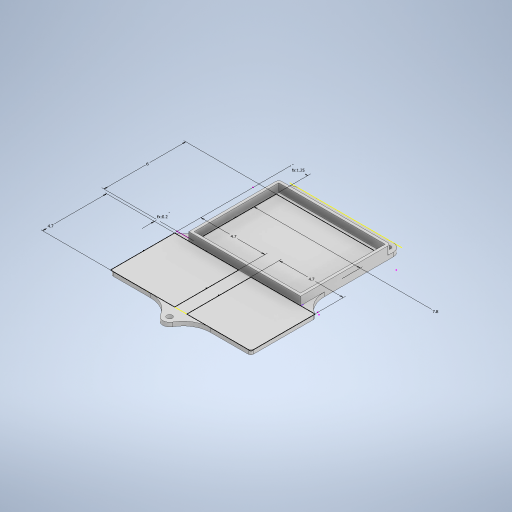
# Autodesk Inventor part: baseCarrito2
Saved by Autodesk Inventor 2024 (Build 280153000, 153)
## iProperties
Created: 2024-04-22
Part Number: baseCarrito2
Material: Generic
Document SubType Name: Modeling
Designer: Ruki
Density: 1 g/cm^3
Appearance: Default
Author: Ruki
Autodesk Inventor part; units mm, degrees
ref_plane "YZ Plane" through (0, 0, 0) normal (1, 0, 0) x (0, 1, 0)
ref_plane "XZ Plane" through (0, 0, 0) normal (0, 1, 0) x (-1, 0, 0)
ref_plane "XY Plane" through (0, 0, 0) normal (0, 0, 1) x (1, 0, 0)
sketch "Sketch1" plane through (0, 0, 0) normal (0, 1, 0) x (-1, 0, 0)
  line L0 (0, 0) -> (-103, 0)
  line L1 (-103, 0) -> (-103, -121)
  line L2 (-103, -121) -> (0, -121)
  line L3 (0, -121) -> (0, 0)
  line L4 (-10.5, -121) -> (-92.5, -121)
  line L5 (-92.5, -121) -> (-92.5, -49)
  line L6 (-92.5, -49) -> (-10.5, -49)
  line L7 (-10.5, -49) -> (-10.5, -121)
  circle A0 centre (-15.5, -116) radius 2
  circle A1 centre (-87.5, -116) radius 2
  line L8 (0, -49) -> (-47, -49)
  line L9 (-47, -49) -> (-47, -2)
  line L10 (-47, -2) -> (0, -2)
  line L11 (0, -2) -> (0, -49)
  line L12 (-56, -49) -> (-103, -49)
  line L13 (-103, -49) -> (-103, -2)
  line L14 (-103, -2) -> (-56, -2)
  line L15 (-56, -2) -> (-56, -49)
  line L16 (-10.5, -49) -> (0, -49)
  line L17 (-92.5, -49) -> (-103, -49)
  circle A2 centre (-51.5, 8) radius 2
  circle A3 centre (-51.5, 8) radius 5
  line L18 (-46.5, 8) -> (-46.5, 0)
  line L19 (-46.5, 0) -> (-56.5, 0)
  line L20 (-56.5, 0) -> (-56.5, 8)
  line L21 (0, -47) -> (-103, -47)
  line L22 (-10.5, -49) -> (-10.5, -47)
  line L23 (-92.5, -49) -> (-92.5, -47)
  point P0 (0, -62)
  point P1 (-103, -62)
  point P2 (-51.5, -121)
  point P3 (-92.5, -121)
  point P4 (-10.5, -121)
  point P5 (0, -25.5)
  point P6 (-47, -25.5)
  point P7 (-56, -25.5)
  point P8 (-51.5, 0)
  point P9 (-56.5, 8)
  point P10 (-56.5, 0)
  point P11 (-46.5, 0)
  point P12 (-46.5, 8)
  dimension "d0" = 121
  dimension "d1" = 103
  dimension "d3" = 82
  dimension "d4" = 72
  dimension "d5" = 10.5
  dimension "d6" = 4
  dimension "d7" = 5
  dimension "d8" = 5
  dimension "d14" = 5
  dimension "d15" = 5
  dimension "d31" = 47
  dimension "d32" = 47
  dimension "d33" = 47
  dimension "d34" = 47
  dimension "d54" = 51.5
  dimension "d55" = 8
  dimension "d56" = 10
  dimension "d61" = 2
  constraints: 48 end point, 10 point on line, 9 parallel, 7 perpendicular, 5 collinear, 5 midpoint, 4 centre point, 4 horizontal, 2 tangent, 1 coincident, 1 equal radius, 1 vertical
  measures "d0" distance of L0.start L2.end
  measures "d1" distance of L1.end L2.end
  measures "d3" distance of L4.end L4.start
  measures "d4" distance from line of L6 point (-51.5, -121)
  measures "d5" distance between parallel lines of L3 L7
  measures "d6" diameter of A0
  measures "d7" distance from line of L2 A0.centre
  measures "d8" distance from line of L7 A0.centre
  measures "d14" distance from line of L4 A1.centre
  measures "d15" distance from line of L5 A1.centre
  measures "d31" distance of L9.end L10.end
  measures "d32" distance of L13.end L14.end
  measures "d33" distance of L12.end L13.end
  measures "d34" distance between parallel lines of L10 L8
  measures "d54" distance from line of L1 A2.centre
  measures "d55" distance of point (-51.5, 0) A2.centre
  measures "d56" diameter of A3
  measures "d61" distance between parallel lines of L21 L8
extrude "Extrusion1" add sketch "Sketch1" along normal blind 3 contours L3 L10 L9 L21 L15 L14 L1 L0 | L0 L20 A3 L18 | L3 L21 L9 L10 | A3 | L22 L6 L9 L21 | L9 L6 L15 L21 | L14 L15 L21 L1 | L7 L2 L5 L6 | L15 L6 L23 L21
sketch "Sketch2" plane through (0, 3, 0) normal (0, 1, 0) x (1, 0, 0)
  line L0 (0, 47) -> (47, 47)
  line L1 (47, 47) -> (47, 0)
  line L2 (47, 0) -> (0, 0)
  line L3 (0, 0) -> (0, 47)
  line L4 (0, 47) -> (0, 0) projected
  line L5 (0, 0) -> (103, 0) projected
  line L6 (56, 47) -> (103, 47)
  line L7 (103, 47) -> (103, 0)
  line L8 (103, 0) -> (56, 0)
  line L9 (56, 0) -> (56, 47)
  line L10 (103, 0) -> (103, 47) projected
  line L11 (92.5, 121) -> (10.5, 121) projected
  line L12 (10.5, 49) -> (0, 49) projected
  line L13 (12.5, 109) -> (90.5, 109)
  line L14 (90.5, 109) -> (90.5, 49)
  line L15 (90.5, 49) -> (12.5, 49)
  line L16 (12.5, 49) -> (12.5, 109)
  line L17 (10.5, 49) -> (10.5, 47)
  line L18 (92.5, 49) -> (92.5, 47)
  point P0 (23.5, 47)
  point P1 (105, 48)
  point P2 (0, 24.5)
  point P3 (10.5, 121)
  point P4 (56, 23.5)
  point P5 (47, 23.5)
  point P6 (0, 104.7)
  point P7 (105, 104.7)
  point P8 (103, 49)
  point P9 (90.5, 79)
  point P10 (12.5, 79)
  dimension "d21" = 47
  dimension "d22" = 47
  dimension "d26" = 47
  dimension "d38" = 2
  dimension "d39" = 78
  dimension "d40" = 60
  dimension "d43" = 12.5
  constraints: 28 end point, 6 parallel, 5 collinear, 5 midpoint, 5 perpendicular, 4 point on line, 3 horizontal, 1 vertical, 2 other
  measures "d21" distance from line of L2 point (23.5, 47)
  measures "d22" distance between parallel lines of L3 L1
  measures "d26" distance between parallel lines of L7 L9
  measures "d38" distance between parallel lines of L12 L0
  measures "d39" distance of point (90.5, 79) point (12.5, 79)
  measures "d40" distance between parallel lines of L15 L13
  measures "d43" distance between parallel lines of L4 L16
sketch "Sketch3" plane through (0, 3, 0) normal (0, 1, 0) x (1, 0, 0)
  line L0 (10.5, 113) -> (92.5, 113)
  line L1 (92.5, 113) -> (92.5, 47)
  line L2 (92.5, 47) -> (10.5, 47)
  line L3 (10.5, 47) -> (10.5, 113)
  line L4 (12.5, 111) -> (90.5, 111)
  line L5 (90.5, 111) -> (90.5, 49)
  line L6 (90.5, 49) -> (12.5, 49)
  line L7 (12.5, 49) -> (12.5, 111)
  line L8 (0, 47) -> (0, 0) projected
  line L9 (0, 0) -> (103, 0) projected
  point P0 (0, 49)
  dimension "d44" = 78
  dimension "d45" = 62
  dimension "d46" = 12.5
  dimension "d47" = 49
  dimension "d48" = 82
  dimension "d49" = 2
  dimension "d51" = 66
  dimension "d52" = 2
  constraints: 16 end point, 4 parallel, 2 horizontal, 2 perpendicular
  measures "d44" distance between parallel lines of L5 L7
  measures "d45" distance between parallel lines of L6 L4
  measures "d46" distance between parallel lines of L8 L7
  measures "d47" distance between parallel lines of L9 L6
  measures "d48" distance between parallel lines of L1 L3
  measures "d49" distance between parallel lines of L3 L7
  measures "d51" distance between parallel lines of L2 L0
  measures "d52" distance between parallel lines of L4 L0
fillet "Fillet1" radius 20 2 edges at (56.5, 1.5, 0) (46.5, 1.5, 0)
extrude "Extrusion2" add sketch "Sketch3" along normal blind 6
fillet "Fillet3" radius 20 2 edges at (92.5, 1.5, -47) (10.5, 1.5, -47)
fillet "Fillet4" radius 6 2 edges at (92.5, 1.5, -121) (10.5, 1.5, -121)
fillet "Fillet5" radius 2 6 edges at (0, 1.5, 0) (103, 1.5, 0) (0, 1.5, -47) (103, 1.5, -47) (92.5, 6, -113) (10.5, 6, -113)
equation "\"d0\" = d34 + d37 + d4"
equation "\"d1\" = 2 * d47 + d36"
equation "\"d5\" = -0.5 * d3 + 0.5 * d1"
equation "\"d54\" = 0.5 * d1"
equation "\"d38\" = d37"
equation "\"d43\" = -0.5 * d39 + 0.5 * d1"
equation "\"d44\" = d39"
equation "\"d46\" = d43"
equation "\"d47\" = d38 + d21"
equation "\"d48\" = d3"
equation "\"d2\" = 0.5 * d0"
equation "\"d37\" = 2"
equation "\"d36\" = 5"
body "Solid1"
